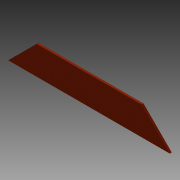
# Autodesk Inventor part: Trapezoid Polycarbonate End Ramp 125
Saved by Autodesk Inventor 2015 (Build 190159000, 159)
## iProperties
Created: 2015-01-20
Part Number: Trapezoid Polycarbonate End Ramp 125
Material: Wood (Oak)
Document SubType Name: Modeling
Designer: Peter
Density: 0.76 g/cm^3
Appearance: White Oak - Natural Medium Gloss
Author: Peter
Autodesk Inventor part; units mm, degrees
ref_plane "YZ Plane" through (0, 0, 0) normal (1, 0, 0) x (0, 1, 0)
ref_plane "XZ Plane" through (0, 0, 0) normal (0, 1, 0) x (-1, 0, 0)
ref_plane "XY Plane" through (0, 0, 0) normal (0, 0, 1) x (1, 0, 0)
sketch "Sketch1" plane through (0, 0, 0) normal (0, 0, 1) x (1, 0, 0)
  line L0 (0, 137.16) -> (508, 137.16)
  line L1 (508, 137.16) -> (645.16, 0)
  line L2 (645.16, 0) -> (0, 0)
  line L3 (0, 137.16) -> (-137.16, 0)
  line L4 (-137.16, 0) -> (0, 0)
  dimension "d0" = 508
  dimension "d1" = 137.16
  dimension "d2" = 137.16
  dimension "d5" = 137.16
  constraints: 10 end point, 1 horizontal, 1 parallel
  measures "d0" distance of L0.start L0.end
  measures "d1" horizontal distance of L1.end L0.end
  measures "d2" distance of L2.end L0.start
  measures "d5" distance of L3.end L2.end
extrude "Extrusion1" add sketch "Sketch1" along normal blind 9.525
body "Solid1"
